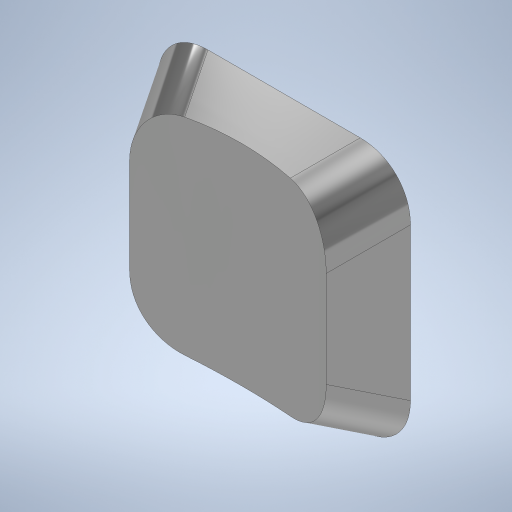
# Autodesk Inventor part: Button_16x16
Saved by Autodesk Inventor 2024 (Build 280153000, 153)
## iProperties
Created: 2023-09-15
Part Number: Button_16x16
Material: 聚丙烯
Document SubType Name: Modeling
Designer: nicx5
Density: 0.899 g/cm^3
Appearance: 铬 - 黑色抛光
Author: nicx5
Autodesk Inventor part; units mm, degrees
ref_plane "YZ Plane" through (0, 0, 0) normal (1, 0, 0) x (0, 1, 0)
ref_plane "XZ Plane" through (0, 0, 0) normal (0, 1, 0) x (-1, 0, 0)
sketch "草图2" plane through (0, 0, 0) normal (0, 0, 1) x (1, 0, 0)
  line L0 (-7, 7) -> (7, 7)
  line L1 (7, 7) -> (7, -7)
  line L2 (7, -7) -> (-7, -7)
  line L3 (-7, -7) -> (-7, 7)
  line L4 (-7, 7) -> (7, -7) construction
  line L5 (7, 7) -> (-7, -7) construction
  point P0 (0, 0)
  dimension "d7" = 14
  dimension "d8" = 14
  constraints: 12 end point, 2 midpoint
  measures "d7" distance of L1.end L2.end
  measures "d8" distance of L0.end L1.end
ref_plane "工作平面1" through (0, 0, -4) normal (0, 0, 1) x (1, 0, 0)
sketch "草图3" plane through (0, 0, -4) normal (0, 0, 1) x (1, 0, 0)
  line L0 (-9, 9) -> (9, 9)
  line L1 (9, 9) -> (9, -9)
  line L2 (9, -9) -> (-9, -9)
  line L3 (-9, -9) -> (-9, 9)
  line L4 (-9, 9) -> (9, -9) construction
  line L5 (9, 9) -> (-9, -9) construction
  point P0 (0, 0)
  point P1 (0, 0)
  dimension "d10" = 18
  dimension "d11" = 18
  constraints: 12 end point, 2 midpoint
  measures "d10" distance of L1.end L2.end
  measures "d11" distance of L0.end L1.end
loft "放样1" add profiles "草图2", "草图3"
fillet "圆角2" radius 4 4 edges at (8, 8, -2) (8, -8, -2) (-8, -8, -2) (-8, 8, -2)
sketch "草图4" plane through (0, 0, 0) normal (0, 1, 0) x (-1, 0, 0)
  arc A0 (-7, 0) -> (7, 0) centre (0, 25.1687) ccw
  line L0 (7, 0) -> (-7, 0)
  point P0 (0, 0)
  point P1 (-7, 0)
  point P2 (7, 0)
  constraints: 2 end point, 2 point on circle, 1 centre point
extrude "拉伸2" cut sketch "草图4" along normal mid plane 16
